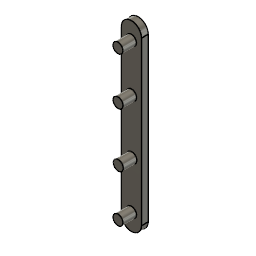
Atlas_Shelf_Truss_ST001 v1.0 (Autodesk Fusion 360 design; units mm, degrees)
part number: 2026-07-26-17-04-48-127
Autodesk Fusion 360 part; units mm, degrees
sketch "Sketch5" plane through (0, 0, 0) normal (0, 0, 1) x (1, 0, 0)
  line L0 (3.81, -34.29) -> (-3.81, -34.29)
  line L1 (-3.81, -34.29) -> (-3.81, 34.29)
  line L2 (-3.81, 34.29) -> (3.81, 34.29)
  line L3 (3.81, 34.29) -> (3.81, -34.29)
  line L4 (3.81, -34.29) -> (-3.81, 34.29) construction
  line L5 (-3.81, -34.29) -> (3.81, 34.29) construction
  dimension "d45" = 7.62
  dimension "d46" = 68.58
  constraint horizontal L0
  constraint perpendicular L0 L1
  constraint parallel L0 L2
  constraint parallel L1 L3
  constraint coincident L4 origin
  constraint coincident L5 origin
  measures "d45" distance of L1.end L2.end
  measures "d46" distance of L0.end L1.end
extrude "Extrude3" add sketch "Sketch5" along normal blind 2.54
fillet "Fillet2" radius 3.81 4 edges at (3.81, 34.29, 1.27) (3.81, -34.29, 1.27) (-3.81, 34.29, 1.27) (-3.81, -34.29, 1.27)
sketch "Sketch6" plane through (0, 0, 2.54) normal (0, 0, 1) x (1, 0, 0)
  arc A0 (-3.81, -30.48) -> (3.81, -30.48) centre (0, -30.48) ccw
  line L0 (3.81, -30.48) -> (3.81, 30.48)
  arc A1 (3.81, 30.48) -> (-3.81, 30.48) centre (0, 30.48) ccw
  line L1 (-3.81, 30.48) -> (-3.81, -30.48)
  circle A2 centre (-0.0028, 27.94) radius 1.905
  circle A3 centre (0.0507, 10.16) radius 1.905
  circle A4 centre (0.1601, -10.16) radius 1.905
  circle A5 centre (0.0346, -27.94) radius 1.905
  point P0 (0.0507, 10.16)
  point P1 (-0.0028, 27.94)
  point P2 (0.1601, -10.16)
  point P3 (0.0346, -27.94)
  dimension "d54" = 10.16
  dimension "d55" = 27.94
  dimension "d56" = 10.16
  dimension "d57" = 27.94
  dimension "d58" = 3.81
  dimension "d59" = 3.81
  dimension "d60" = 3.81
  dimension "d61" = 3.81
  constraint coincident P1 A2.centre
  constraint coincident P0 A3.centre
  constraint coincident P2 A4.centre
  constraint coincident P3 A5.centre
  measures "d54" vertical distance of origin A3.centre
  measures "d55" vertical distance of origin P1
  measures "d56" vertical distance of origin P2
  measures "d57" vertical distance of origin P3
  measures "d58" diameter of A2
  measures "d59" diameter of A3
  measures "d60" diameter of A4
  measures "d61" diameter of A5
extrude "Extrude4" add sketch "Sketch6" along normal blind 5.08 contours A2 | A3 | A4 | A5
equation "shelfThickness = 0.1 in"
equation "shelfWidth = 1.5 in"
equation "shelfDepth = 1.5 in"
equation "trussThickness = 0.1 in"
equation "tabInset = trussThickness / 2"
equation "tabWidth = 0.5 in"
equation "tab1Offset = tabBaseOffset + tabWidth / 2"
equation "tab2Offset = tabBaseOffset + ( tabWidth / 2 ) + tabSeparation"
equation "tabBaseOffset = 0.15 in"
equation "tabSeparation = tabWidth + 0.2 in"
equation "trussWidth = 0.3 in"
equation "trussLength = ( 2 * tab2Offset + 0.5 in )"
equation "d45 = trussWidth"
equation "d46 = trussLength"
equation "d47 = trussThickness"
equation "tabHeight = 0.3 in"
equation "studLength = 0.2 in"
equation "studDiameter = 0.15 in"
equation "d54 = tab1Offset"
equation "d55 = tab2Offset"
equation "d56 = tab1Offset"
equation "d57 = tab2Offset"
equation "d58 = studDiameter"
equation "d59 = studDiameter"
equation "d60 = studDiameter"
equation "d61 = studDiameter"
equation "d62 = studLength"
